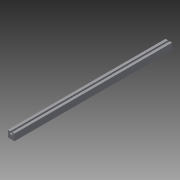
# Autodesk Inventor part: rail
Saved by Autodesk Inventor 2015 (Build 190159000, 159)
## iProperties
Created: 2015-04-09
Part Number: rail
Material: Generic
Document SubType Name: Modeling
Designer: WASHHSST
Density: 1 g/cm^3
Appearance: Default
Author: WASHHSST
Autodesk Inventor part; units mm, degrees
ref_plane "YZ Plane" through (0, 0, 0) normal (1, 0, 0) x (0, 1, 0)
ref_plane "XZ Plane" through (0, 0, 0) normal (0, 1, 0) x (-1, 0, 0)
ref_plane "XY Plane" through (0, 0, 0) normal (0, 0, 1) x (1, 0, 0)
sketch "Sketch1" plane through (0, 0, 0) normal (0, 0, 1) x (1, 0, 0)
  line L0 (0, 0) -> (50.8, 0)
  line L1 (50.8, 0) -> (50.8, 50.8)
  line L2 (50.8, 50.8) -> (0, 50.8)
  line L3 (0, 50.8) -> (0, 0)
  line L4 (19.05, 50.8) -> (19.05, 38.1)
  line L5 (19.05, 38.1) -> (12.7, 38.1)
  line L6 (12.7, 38.1) -> (12.7, 31.75)
  line L7 (12.7, 31.75) -> (38.1, 31.75)
  line L8 (38.1, 31.75) -> (38.1, 38.1)
  line L9 (38.1, 38.1) -> (31.75, 38.1)
  line L10 (31.75, 38.1) -> (31.75, 50.8)
  dimension "d0" = 50.8
  dimension "d1" = 50.8
  dimension "d2" = 19.05
  dimension "d3" = 19.05
  dimension "d4" = 12.7
  dimension "d5" = 12.7
  dimension "d6" = 6.35
  dimension "d7" = 6.35
  dimension "d8" = 6.35
  constraints: 22 end point, 6 perpendicular, 4 point on line, 2 parallel, 1 horizontal, 1 vertical
  measures "d0" distance of L2.end L1.end
  measures "d1" distance of L1.end L0.end
  measures "d2" distance between parallel lines of L3 L4
  measures "d3" distance between parallel lines of L1 L10
  measures "d4" distance between parallel lines of L4 L10
  measures "d5" distance between parallel lines of L2 L9
  measures "d6" distance between parallel lines of L4 L6
  measures "d7" distance between parallel lines of L10 L8
  measures "d8" distance between parallel lines of L9 L7
extrude "Extrusion1" add sketch "Sketch1" along normal blind 1219.2 contours L3 L2 L4 L5 L6 L7 L8 L9 L10 L1 L0
body "Solid1"
